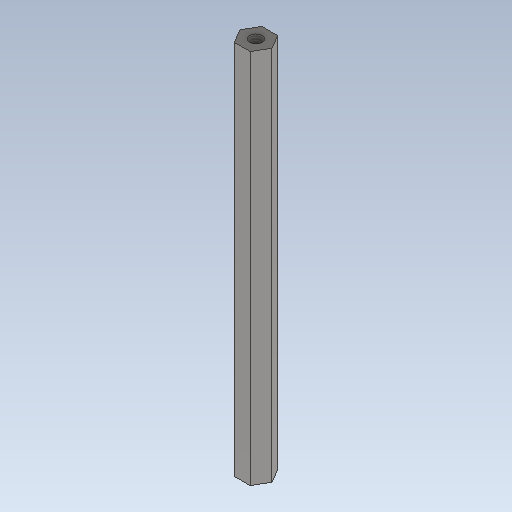
# Autodesk Inventor part: ASU-375H
Saved by Autodesk Inventor 2020.4 (Build 244396000, 396)
## iProperties
Created: 2021-09-09
Part Number: ASU-375H
Material: アルミニウム 2014-T4
Document SubType Name: Modeling
Designer: Masato
Density: 2.8 g/cm^3
Appearance: 半つや出し
Mass: 4.68169 g
Surface Area: 14.0257 cm^2
Volume: 1.67203 cm^3
Description: 既製品
Author: Masato Kubotera
Autodesk Inventor part; units mm, degrees
ref_plane "YZ Plane" through (0, 0, 0) normal (1, 0, 0) x (0, 1, 0)
ref_plane "XZ Plane" through (0, 0, 0) normal (0, 1, 0) x (-1, 0, 0)
ref_plane "XY Plane" through (0, 0, 0) normal (0, 0, 1) x (1, 0, 0)
sketch "スケッチ1" plane through (0, 0, 0) normal (0, 0, 1) x (1, 0, 0)
  line L0 (0, 37.5) -> (0, -37.5)
  line L1 (0, -37.5) -> (4.7631, -37.5)
  line L2 (4.7631, -37.5) -> (4.7631, 37.5)
  line L3 (4.7631, 37.5) -> (0, 37.5)
  point P0 (0, 0)
  point P1 (0, 0)
  dimension "d0" = 75
  dimension "d1" = 4.7631
  constraints: 8 end point, 3 perpendicular, 1 coincident, 1 midpoint, 1 vertical
  measures "d0" distance of L0.start L0.end
  measures "d1" distance from line of L0.start L2
revolve "回転1" add sketch "スケッチ1" angle 360 about axis through (0, 37.5, 0) along (0, -1, 0)
sketch "スケッチ2" plane through (0, 37.5, 0) normal (0, 1, 0) x (1, 0, 0)
  line L0 (3.1754, 0) -> (1.5877, -2.75)
  line L1 (1.5877, -2.75) -> (-1.5877, -2.75)
  line L2 (-1.5877, -2.75) -> (-3.1754, 0)
  line L3 (-3.1754, 0) -> (-1.5877, 2.75)
  line L4 (-1.5877, 2.75) -> (1.5877, 2.75)
  line L5 (1.5877, 2.75) -> (3.1754, 0)
  circle A0 centre (0, 0) radius 4.7631
  point P0 (0, 0)
  dimension "d3" = 5.5
  constraints: 12 end point, 2 coincident, 1 centre point
  measures "d3" distance between parallel lines of L4 L1
extrude "押し出し1" cut sketch "スケッチ2" against normal through all
hole "穴1" at (0, 37.5, 0) direction (0, -1, 0) diameter 2.459 depth 6 thread size "M3x0.5" class "6H" standard "ISO Metric profile"
sketch "スケッチ3" plane through (-1.5877, -37.5, 2.75) normal (0, -1, 0) x (1, 0, 0)
  point P0 (1.5877, -2.75)
  point P1 (1.5877, -2.75)
  constraints: 1 coincident
hole "穴2" at (0, -37.5, 0) direction (0, 1, 0) diameter 2.459 depth 6 thread size "M3x0.5" class "6H" standard "ISO Metric profile"
